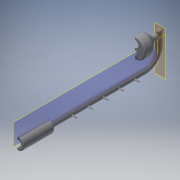
# Autodesk Inventor part: lampa_nadrazni
Saved by Autodesk Inventor 2018 (Build 220112000, 112)
## iProperties
Created: 2018-12-13
Part Number: lampa_nadrazni
Material: Generic
Document SubType Name: Modeling
Designer: petal
Density: 1 g/cm^3
Appearance: Default
Author: petal
Autodesk Inventor part; units mm, degrees
ref_plane "YZ Plane" through (0, 0, 0) normal (1, 0, 0) x (0, 1, 0)
ref_plane "XZ Plane" through (0, 0, 0) normal (0, 1, 0) x (-1, 0, 0)
ref_plane "XY Plane" through (0, 0, 0) normal (0, 0, 1) x (1, 0, 0)
sketch "Sketch1" plane through (0, 0, 0) normal (0, 0, 1) x (1, 0, 0)
  line L0 (0, 0) -> (0, 160)
  line L1 (0, 160) -> (4, 160) construction
  line L2 (4, 160) -> (4, 40)
  line L3 (0, 0) -> (8, 0)
  line L4 (8, 0) -> (8, 40)
  line L5 (8, 40) -> (4, 40)
  line L6 (4.125, 1.5) -> (4.5, 1.5)
  line L7 (4.5, 1.5) -> (4.5, 0)
  line L8 (4.125, 1.5) -> (4.125, 5.5)
  line L9 (4.125, 5.5) -> (6.5, 5.5)
  line L10 (6.5, 5.5) -> (6.5, 38.5)
  line L11 (6.5, 38.5) -> (2.5, 38.5)
  line L12 (2.5, 160) -> (4, 160)
  line L13 (4.125, 5.5) -> (4.125, 5.5)
  line L14 (4.125, 5.5) -> (6.5, 5.5)
  line L15 (2.5, 38.5) -> (2.5, 160)
  dimension "d0" = 160
  dimension "d3" = 8
  dimension "d4" = 40
  dimension "d20" = 1.5
  dimension "d22" = 1.5
  dimension "d26" = 1.5
  dimension "d27" = 4
  dimension "d29" = 9
  dimension "d73" = 8.25
  dimension "d74" = 8.25
  dimension "d75" = 0
  dimension "d78" = 5
  dimension "d79" = 1.5
  constraints: 32 end point, 6 perpendicular, 5 vertical, 4 point on line, 3 horizontal, 1 collinear, 1 parallel
  measures "d0" distance of L0.start L0.end
  measures "d3" distance of L0.start L3.end
  measures "d4" distance of L3.end L4.end
  measures "d20" distance between parallel lines of L4 L10
  measures "d22" distance between parallel lines of L5 L11
  measures "d26" distance from line of L3.end L6
  measures "d27" distance of L8.end L6.start
  measures "d29" diameter of L7 L0
  measures "d73" diameter of L8 L0
  measures "d74" diameter of L13 L0
  measures "d75" distance between parallel lines of L9 L14
  measures "d78" diameter of L15 L0
  measures "d79" distance between parallel lines of L15 L2
revolve "Revolution1" add sketch "Sketch1" angle 360 about axis through (0, 0, 0) along (0, 1, 0)
fillet "Fillet1" radius 2 1 edges at (-8, 40, 0)
fillet "Fillet2" radius 1 1 edges at (-8, 0, 0)
sketch "Sketch17" plane through (0, 160, 0) normal (0, 1, 0) x (1, 0, 0)
  circle A0 centre (0, 0) radius 2.5 projected
  circle A1 centre (0, 0) radius 4 projected
sketch "Sketch18" plane through (0, 0, 0) normal (1, 0, 0) x (0, 1, 0)
  line L0 (160, 2.5) -> (160, -2.5) projected
  arc A0 (160, 0) -> (180, 20) centre (160, 20) ccw
  line L1 (180, 20) -> (180, 35)
  point P0 (0, 0)
  dimension "d80" = 20
  dimension "d81" = 20
  dimension "d82" = 15
  constraints: 2 end point, 2 point on circle, 1 centre point, 1 midpoint, 1 vertical
  measures "d80" radius of A0
  measures "d81" distance from line of L1.end L0
  measures "d82" vertical distance of L1.end A0.centre
sweep "Sweep2" add profiles "Sketch17" path "Sketch18" path curves A0 L1
ref_plane "Work Plane6" through (0, 180, 30) normal (0, 0, 1) x (1, 0, 0)
sketch "Sketch19" plane through (0, 180, 30) normal (0, 0, 1) x (1, 0, 0)
  circle A0 centre (0, 0) radius 4 construction
  circle A1 centre (0, 0) radius 2.5 construction
  line L0 (-2.5, -20) -> (-2.5, 0) construction
  line L1 (-4, -9.822747) -> (-4, 0)
  line L2 (-4, -9.822747) -> (-13, -18.822747)
  line L3 (-13, -18.822747) -> (-13, -27.822747)
  line L4 (-2.5, 0) -> (-2.5, -10.444067)
  line L5 (-2.5, -10.444067) -> (-11.5, -19.444067)
  line L6 (-11.5, -19.444067) -> (-11.5, -27.822747)
  line L7 (-4, 0) -> (-2.5, 0)
  line L8 (-13, -27.822747) -> (-11.5, -27.822747)
  line L9 (0, 0) -> (0, -10.328102)
  point P0 (0, -180)
  dimension "d87" = 9.82275
  dimension "d88" = 9
  dimension "d89" = 9
  dimension "d90" = 9
  constraints: 18 end point, 3 vertical, 2 horizontal alignment, 1 horizontal, 1 parallel, 1 point on line, 3 other
  measures "d87" distance of L1.end L1.start
  measures "d88" horizontal distance of L2.end L1.start
  measures "d89" distance of L2.end L3.end
  measures "d90" horizontal distance of L2.end L1.start
revolve "Revolution4" add sketch "Sketch19" angle 360 about axis through (0, 180, 30) along (0, -1, 0)
sketch "Sketch20" plane through (0, 180, 35) normal (0, 0, 1) x (1, 0, 0)
  circle A0 centre (0, 0) radius 2.5 projected
  circle A1 centre (0, 0) radius 4 projected
  point P0 (0, -180)
extrude "Extrusion10" add sketch "Sketch20" along normal blind 2 contours A0 | A1
sketch "Sketch21" plane through (0, 152.177253, 30) normal (0, -1, 0) x (1, 0, 0)
  circle A0 centre (0, 0) radius 11.5 projected
  circle A1 centre (0, 0) radius 13 projected
  circle A2 centre (0, -5) radius 2.75
  circle A3 centre (0, 5) radius 4.5
  point P0 (0, -30)
  dimension "d94" = 5
  dimension "d95" = 5
  dimension "d96" = 5.5
  dimension "d97" = 9
  constraints: 2 centre point
  measures "d94" distance of A2.centre A0.centre
  measures "d95" distance of A0.centre A3.centre
  measures "d96" diameter of A2
  measures "d97" diameter of A3
extrude "Extrusion11" add sketch "Sketch21" along normal blind 2 contours A0 | A1
sketch "Sketch25" plane through (0, 150.177253, 30) normal (0, -1, 0) x (1, 0, 0)
  arc A0 (-2.5, 0) -> (2.5, 0) centre (0, 0) ccw construction
  circle A1 centre (0, 0) radius 11.5
  circle A2 centre (0, 5) radius 4.5 construction
  circle A3 centre (0, -5) radius 2.75 construction
  circle A4 centre (0, 0) radius 13 projected
  point P0 (0, -30)
  dimension "d122" = 1.5
  constraints: 1 centre point, 1 coincident
  measures "d122" radial gap between concentric circles of A4 A1
extrude "Extrusion15" add sketch "Sketch25" along normal blind 2
sketch "Sketch11" plane through (0, 0, 0) normal (1, 0, 0) x (0, 1, 0)
  line L0 (184.940596, 50.492575) -> (0, 50.492575)
  line L1 (0, 50.492575) -> (0, -25.115985)
  line L2 (0, -25.115985) -> (184.940596, -25.115985)
  line L3 (184.940596, -25.115985) -> (184.940596, 50.492575)
  point P0 (0, 0)
  constraints: 8 end point, 2 parallel, 1 horizontal, 1 perpendicular
extrude "Extrusion4" cut sketch "Sketch11" against normal blind 20
fillet "Fillet7" radius 5 2 edges at (4, 170.1773, 30) (13, 161.1773, 30)
fillet "Fillet7" radius 2 3 edges at (4, 180, 37) (2.8284, 177.1716, 27.1716) (2.8284, 177.1716, 32.8284)
fillet "Fillet7" radius 2 1 edges at (13, 148.1773, 30)
ref_plane "Work Plane7" through (0, 176, 20) normal (0, -1, 0) x (1, 0, 0)
sketch "Sketch22" plane through (0, 176, 20) normal (0, -1, 0) x (1, 0, 0)
  line L0 (0, 12.5) -> (0, 7.5)
  spline S0 degree 6 poles (0, 7.5) (0.182885, 7.5) (0.364262, 7.516055) (0.541387, 7.547667) (0.711601, 7.593516) (0.872474, 7.651467) (1.136801, 7.76986) (1.24574, 7.826986) (1.348778, 7.889034) (1.446008, 7.955374) (1.537562, 8.025487) (1.716501, 8.17831) (1.803043, 8.261645) (1.883418, 8.348485) (1.957825, 8.438488) (2.026424, 8.531421) (2.156101, 8.728773) (2.216486, 8.833599) (2.270471, 8.941275) (2.318043, 9.051519) (2.35916, 9.164102) (2.428795, 9.395243) (2.45714, 9.513919) (2.478522, 9.634257) (2.492831, 9.755712) (2.5, 9.877788) (2.5, 10.122791) (2.492763, 10.245443) (2.478319, 10.367466) (2.456735, 10.488355) (2.428124, 10.607561) (2.358176, 10.838584) (2.31714, 10.950566) (2.269714, 11.060227) (2.215939, 11.167343) (2.155826, 11.271637) (2.001861, 11.505973) (1.903327, 11.633738) (1.793486, 11.755721) (1.67181, 11.871234) (1.537672, 11.979121) (1.285785, 12.147705) (1.174208, 12.21321) (1.055841, 12.273228) (0.930832, 12.326827) (0.799425, 12.373023) (0.557807, 12.439369) (0.449978, 12.463169) (0.339355, 12.481473) (0.226856, 12.493825) (0.113424, 12.5) (0, 12.5) knots 0 0 0 0 0 0 0 0.1142659 0.1142659 0.1142659 0.1142659 0.1142659 0.20209213 0.20209213 0.20209213 0.20209213 0.20209213 0.29696097 0.29696097 0.29696097 0.29696097 0.29696097 0.39770415 0.39770415 0.39770415 0.39770415 0.39770415 0.49990013 0.49990013 0.49990013 0.49990013 0.49990013 0.60258035 0.60258035 0.60258035 0.60258035 0.60258035 0.70282594 0.70282594 0.70282594 0.70282594 0.70282594 0.83484694 0.83484694 0.83484694 0.83484694 0.83484694 0.9288037 0.9288037 0.9288037 0.9288037 0.9288037 1 1 1 1 1 1 1
  point P0 (0, -20)
  constraints: 1 vertical alignment
extrude "Extrusion12" cut sketch "Sketch22" against normal blind 4
sketch "Sketch23" plane through (0, 180, 35) normal (0, 0, -1) x (-1, 0, 0)
  line L0 (0, -2.5) -> (0, 2.5) projected
  arc A0 (0, 2.5) -> (0, -2.5) centre (0, 0) ccw projected
  point P0 (0, -180)
extrude "Extrusion13" cut sketch "Sketch23" along normal blind 10
fillet "Fillet8" radius 1 5 edges at (1.7678, 178.2322, 28.2322) (1.7678, 178.2322, 31.7678) (2.5, 169.5559, 30) (11.5, 160.5559, 30) (2.5, 180, 35)
ref_plane "Work Plane8" through (3, 0, 0) normal (-1, 0, 0) x (0, 0, 1)
sketch "Sketch24" plane through (3, 0, 0) normal (-1, 0, 0) x (0, 0, 1)
  line L0 (-2.5, 160) -> (-2.5, 38.5) construction
  line L1 (-2.5, 38.5) -> (2.5, 38.5) construction
  line L2 (2.5, 38.5) -> (2.5, 160) construction
  line L3 (-2.5, 160) -> (2.5, 160) construction
  line L4 (0, 160) -> (0, 38.5)
  circle A0 centre (0, 146) radius 0.75
  circle A1 centre (0, 126) radius 0.75
  circle A2 centre (0, 106) radius 0.75
  circle A3 centre (0, 86) radius 0.75
  circle A4 centre (0, 66) radius 0.75
  point P0 (0, 0)
  dimension "d109" = 1.5
  dimension "d110" = 14
  dimension "d113" = 20
  constraints: 5 centre point, 2 end point, 2 midpoint, 1 point on line, 1 vertical, 8 other
  measures "d109" diameter of A0
  measures "d110" distance from line of L3 A0.centre
  measures "d113" distance of A0.centre A1.centre
extrude "Extrusion14" add sketch "Sketch24" against normal blind 7
fillet "Fillet9" radius 0.5 5 edges at (10, 66, -0.75) (10, 86, -0.75) (10, 106, -0.75) (10, 126, -0.75) (10, 146, -0.75)
equation "\"d22\" = d20"
equation "\"d95\" = d94"
body "Solid1"
